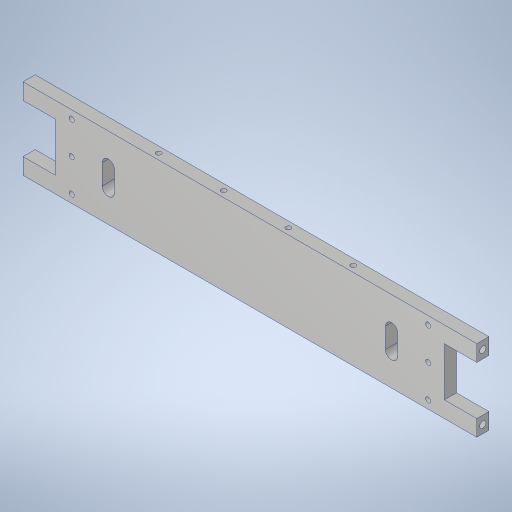
# Autodesk Inventor part: EL2-003
Saved by Autodesk Inventor 2023.4 (Build 274418000, 418)
## iProperties
Created: 2025-01-10
Part Number: EL2-003
Material: Aluminum 6061
Document SubType Name: Modeling
Designer: mavericks
Density: 2.7 g/cm^3
Appearance: Aluminum - Flat
Author: mavericks
Autodesk Inventor part; units mm, degrees
ref_plane "YZ Plane" through (0, 0, 0) normal (1, 0, 0) x (0, 1, 0)
ref_plane "XZ Plane" through (0, 0, 0) normal (0, 1, 0) x (-1, 0, 0)
ref_plane "XY Plane" through (0, 0, 0) normal (0, 0, 1) x (1, 0, 0)
sketch "Sketch1" plane through (0, 0, 0) normal (0, 0, 1) x (1, 0, 0)
  line L0 (-177.8, -31.75) -> (177.8, -31.75)
  line L1 (177.8, -31.75) -> (177.8, 31.75)
  line L2 (177.8, 31.75) -> (-177.8, 31.75)
  line L3 (-177.8, 31.75) -> (-177.8, -31.75)
  line L4 (-177.8, -31.75) -> (177.8, 31.75) construction
  line L5 (177.8, -31.75) -> (-177.8, 31.75) construction
  point P0 (0, 0)
  dimension "d0" = 355.6
  dimension "d1" = 63.5
  constraints: 12 end point, 2 midpoint, 2 parallel, 1 horizontal, 1 perpendicular
  measures "d0" distance of L2.end L1.end
  measures "d1" distance of L1.end L0.end
extrude "Extrusion1" add sketch "Sketch1" along normal blind 9.525
sketch "Sketch4" plane through (0, 0, 9.525) normal (0, 0, 1) x (1, 0, 0)
  line L0 (-139.7, 0) -> (139.7, 0) construction
  point P0 (0, 0)
  point P1 (-139.7, 25.4)
  point P2 (-139.7, -25.4)
  point P3 (139.7, 25.4)
  point P4 (139.7, -25.4)
  point P5 (0, 0)
  dimension "d19" = 25.4
  dimension "d20" = 25.4
  dimension "d21" = 279.4
  constraints: 4 horizontal alignment, 4 vertical alignment, 2 end point, 1 coincident, 1 horizontal, 1 midpoint
  measures "d19" distance of L0.start point (-139.7, 25.4)
  measures "d20" distance of point (-139.7, -25.4) L0.start
  measures "d21" distance of L0.start L0.end
hole "Hole2" at (-139.7, 25.4, 9.525) at (-139.7, 0, 9.525) at (-139.7, -25.4, 9.525) at (139.7, 25.4, 9.525) at (139.7, 0, 9.525) at (139.7, -25.4, 9.525) direction (0, 0, -1) diameter 3.9624 end through all thread size "10-32 UNF" class "2B" standard "ANSI Unified Screw Threads"
sketch "Sketch5" plane through (177.8, -31.75, 0) normal (1, 0, 0) x (0, 0, -1)
  line L0 (0, 63.5) -> (-9.525, 63.5) construction
  line L1 (-4.7625, 57.15) -> (-4.7625, 6.35) construction
  line L2 (0, 0) -> (0, 63.5) construction
  point P0 (0, 31.75)
  point P1 (-4.7625, 63.5)
  point P2 (-4.7625, 31.75)
  point P3 (0, 31.75)
  dimension "d29" = 50.8
  constraints: 3 midpoint, 2 end point, 2 vertical alignment, 1 horizontal alignment, 1 vertical
  measures "d29" distance of L1.start L1.end
hole "Hole3" at (177.8, 25.4, 4.7625) at (177.8, -25.4, 4.7625) direction (-1, 0, 0) diameter 4.9784 depth 25.4 tip angle 118 thread size "1/4-20 UNC" class "2B" standard "ANSI Unified Screw Threads"
sketch "Sketch6" plane through (-177.8, -31.75, 0) normal (-1, 0, 0) x (0, 0, 1)
  line L0 (0, 63.5) -> (9.525, 63.5) construction
  line L1 (4.7625, 57.15) -> (4.7625, 6.35) construction
  point P0 (0, 31.75)
  point P1 (4.7625, 63.5)
  point P2 (4.7625, 31.75)
  dimension "d37" = 50.8
  constraints: 2 end point, 2 midpoint, 2 vertical alignment, 1 horizontal alignment, 1 vertical
  measures "d37" distance of L1.start L1.end
hole "Hole4" at (-177.8, 25.4, 4.7625) at (-177.8, -25.4, 4.7625) direction (1, 0, 0) diameter 4.3434 depth 25.4 tip angle 118 thread size "12-24 UNC" class "2B" standard "ANSI Unified Screw Threads"
sketch "Sketch8" plane through (0, 0, 9.525) normal (0, 0, 1) x (1, 0, 0)
  line L0 (-152.4, 19.05) -> (-177.8, 19.05)
  line L1 (-177.8, 19.05) -> (-177.8, -19.05)
  line L2 (-177.8, -19.05) -> (-152.4, -19.05)
  line L3 (-152.4, -19.05) -> (-152.4, 19.05)
  line L4 (-152.4, 19.05) -> (-177.8, -19.05) construction
  line L5 (-177.8, 19.05) -> (-152.4, -19.05) construction
  line L6 (177.8, 31.75) -> (-177.8, 31.75) projected
  line L7 (-177.8, 31.75) -> (-177.8, -31.75) projected
  line L8 (177.8, 19.05) -> (152.4, 19.05)
  line L9 (152.4, 19.05) -> (152.4, -19.05)
  line L10 (152.4, -19.05) -> (177.8, -19.05)
  line L11 (177.8, -19.05) -> (177.8, 19.05)
  line L12 (177.8, 19.05) -> (152.4, -19.05) construction
  line L13 (152.4, 19.05) -> (177.8, -19.05) construction
  line L14 (177.8, -31.75) -> (177.8, 31.75) projected
  point P0 (0, 0)
  point P1 (-165.1, 0)
  point P2 (165.1, 0)
  dimension "d45" = 25.4
  dimension "d46" = 38.1
  dimension "d47" = 12.7
  dimension "d49" = 25.4
  dimension "d50" = 38.1
  dimension "d52" = 12.7
  constraints: 24 end point, 4 midpoint, 4 parallel, 2 horizontal, 2 perpendicular, 2 point on line
  measures "d45" distance of L2.end L1.end
  measures "d46" distance of L0.end L1.end
  measures "d47" distance between parallel lines of L6 L0
  measures "d49" distance of L10.end L9.end
  measures "d50" distance of L9.end L8.end
  measures "d52" distance between parallel lines of L6 L8
extrude "Extrusion3" cut sketch "Sketch8" against normal blind 39.6875
sketch "Sketch9" plane through (0, 0, 9.525) normal (0, 0, 1) x (1, 0, 0)
  line L0 (110.998, 7.9375) -> (110.998, -7.9375) construction
  line L1 (106.2355, 7.9375) -> (106.2355, -7.9375)
  line L2 (115.7605, -7.9375) -> (115.7605, 7.9375)
  arc A0 (115.7605, 7.9375) -> (106.2355, 7.9375) centre (110.998, 7.9375) ccw
  arc A1 (106.2355, -7.9375) -> (115.7605, -7.9375) centre (110.998, -7.9375) ccw
  line L3 (-152.4, -19.05) -> (-177.8, -19.05) construction
  line L4 (-177.8, -19.05) -> (-177.8, -31.75) construction
  line L5 (-177.8, -31.75) -> (177.8, -31.75) construction
  line L6 (177.8, -31.75) -> (177.8, -19.05) construction
  line L7 (177.8, -19.05) -> (152.4, -19.05) construction
  line L8 (152.4, -19.05) -> (152.4, 19.05) construction
  line L9 (152.4, 19.05) -> (177.8, 19.05) construction
  line L10 (177.8, 19.05) -> (177.8, 31.75) construction
  line L11 (177.8, 31.75) -> (-177.8, 31.75) construction
  line L12 (-177.8, 31.75) -> (-177.8, 19.05) construction
  line L13 (-177.8, 19.05) -> (-152.4, 19.05) construction
  line L14 (-152.4, 19.05) -> (-152.4, -19.05) construction
  circle A2 centre (139.7, 0) radius 1.9812 construction
  circle A3 centre (-139.7, -25.4) radius 1.9812 construction
  circle A4 centre (-139.7, 25.4) radius 1.9812 construction
  circle A5 centre (-139.7, 0) radius 1.9812 construction
  circle A6 centre (139.7, 25.4) radius 1.9812 construction
  circle A7 centre (139.7, -25.4) radius 1.9812 construction
  line L15 (0, 0) -> (0, 31.75) construction
  line L16 (-110.998, 7.9375) -> (-110.998, -7.9375) construction
  line L17 (-106.2355, 7.9375) -> (-106.2355, -7.9375)
  line L18 (-115.7605, -7.9375) -> (-115.7605, 7.9375)
  arc A8 (-106.2355, 7.9375) -> (-115.7605, 7.9375) centre (-110.998, 7.9375) ccw
  arc A9 (-115.7605, -7.9375) -> (-106.2355, -7.9375) centre (-110.998, -7.9375) ccw
  line L19 (-177.8, -31.75) -> (-177.8, -19.05) construction
  line L20 (-177.8, -19.05) -> (-152.4, -19.05) construction
  line L21 (-152.4, -19.05) -> (-152.4, 19.05) construction
  line L22 (-152.4, 19.05) -> (-177.8, 19.05) construction
  circle A10 centre (-139.7, 0) radius 1.9812 construction
  circle A11 centre (-139.7, -25.4) radius 1.9812 construction
  point P0 (110.998, 0)
  point P1 (110.998, -12.7)
  point P2 (110.998, 12.7)
  point P3 (-110.998, 0)
  point P4 (-110.998, -12.7)
  point P5 (-110.998, 12.7)
  dimension "d55" = 9.525
  dimension "d56" = 25.4
  dimension "d57" = 66.802
  constraints: 26 end point, 12 symmetric about line, 10 point on circle, 6 centre point, 4 tangent, 2 midpoint, 1 horizontal alignment, 1 parallel, 1 vertical, 4 other
  measures "d55" diameter of A1
  measures "d56" distance of point (110.998, -12.7) point (110.998, 12.7)
  measures "d57" horizontal distance of L5.end point (110.998, 0)
extrude "Extrusion4" cut sketch "Sketch9" against normal through all
sketch "Sketch10" plane through (-177.8, 31.75, 0) normal (0, 1, 0) x (1, 0, 0)
  line L0 (355.6, 0) -> (0, 0) construction
  line L1 (0, 0) -> (0, -9.525) construction
  line L2 (355.6, -9.525) -> (0, -9.525) construction
  line L3 (355.6, 0) -> (355.6, -9.525) construction
  line L4 (0, 0) -> (0, -9.525) construction
  line L5 (177.8, 0) -> (177.8, -9.525) construction
  line L6 (0, -9.525) -> (355.6, -9.525) construction
  point P0 (101.6, -4.7625)
  point P1 (152.4, -4.7625)
  point P2 (0, -4.7625)
  point P3 (0, -4.7625)
  point P4 (254, -4.7625)
  point P5 (203.2, -4.7625)
  dimension "d60" = 101.6
  dimension "d61" = 50.8
  constraints: 3 midpoint, 2 end point, 2 horizontal alignment, 2 symmetric about line
  measures "d60" distance of point (0, -4.763) point (101.6, -4.763)
  measures "d61" distance of point (152.4, -4.763) point (101.6, -4.763)
hole "Hole5" at (-76.2, 31.75, 4.7625) at (-25.4, 31.75, 4.7625) at (76.2, 31.75, 4.7625) at (25.4, 31.75, 4.7625) direction (0, -1, 0) diameter 3.9624 end through all thread size "10-32 UNF" class "2B" standard "ANSI Unified Screw Threads"
body "Solid1"
